J3 (Autodesk Fusion 360 design; units mm, degrees)
part number: 2026-06-01-05-43-44-829
Autodesk Fusion 360 part; units mm, degrees
sketch "Sketch1" plane through (0, 0, 0) normal (0, 0, 1) x (1, 0, 0)
  line L0 (0, 0) -> (50, 0)
  line L1 (50, 0) -> (50, 10)
  line L2 (50, 10) -> (0, 10)
  line L3 (0, 10) -> (0, 0)
  dimension "d1" = 50
  dimension "d2" = 10
  constraint horizontal L0
  constraint vertical L1
  constraint horizontal L2
  constraint vertical L3
  constraint coincident L0.start L3.end
  measures "d1" distance of L0.start L0.end
  measures "d2" distance of L0.start L2.end
extrude "Extrude1" add sketch "Sketch1" along normal blind 10
sketch "Sketch2" plane through (0, 0, 10) normal (0, 0, 1) x (-1, 0, 0)
  line L0 (0, -10) -> (0, 0)
  line L1 (0, 0) -> (-50, 0)
  line L2 (-50, 0) -> (-50, -10)
  line L3 (-50, -10) -> (0, -10)
  circle A0 centre (-5, -5) radius 4.5
  circle A1 centre (-25, -5) radius 4.5
  dimension "d5" = 9
  dimension "d6" = 9
  measures "d5" diameter of A0
  measures "d6" diameter of A1
extrude "Extrude2" cut sketch "Sketch2" against normal blind 11 contours A0 | A1
sketch "Sketch3" plane through (50, 0, 0) normal (1, 0, 0) x (0, 1, 0)
  line L0 (0, 0) -> (10, 0)
  line L1 (10, 0) -> (10, 10)
  line L2 (10, 10) -> (0, 10)
  line L3 (0, 10) -> (0, 0)
  circle A0 centre (5, 5) radius 4
  dimension "d9" = 8
  measures "d9" diameter of A0
extrude "Extrude3" cut sketch "Sketch3" against normal blind 3 contours A0
sketch "Sketch4" plane through (0, 0, 0) normal (0, -1, 0) x (1, 0, 0)
  line L0 (0, 0) -> (50, 0)
  line L1 (50, 0) -> (50, 10)
  line L2 (50, 10) -> (0, 10)
  line L3 (0, 10) -> (0, 0)
  circle A0 centre (15, 5) radius 4.5
  circle A1 centre (35, 5) radius 4.5
  dimension "d12" = 9
  dimension "d13" = 9
  measures "d12" diameter of A0
  measures "d13" diameter of A1
extrude "Extrude4" cut sketch "Sketch4" against normal blind 20 contours A0 | A1
sketch "Sketch5" plane through (0, 0, 0) normal (-1, 0, 0) x (0, -1, 0)
  line L0 (-10, 0) -> (0, 0)
  line L1 (0, 0) -> (0, 10)
  line L2 (0, 10) -> (-10, 10)
  line L3 (-10, 10) -> (-10, 0)
  circle A0 centre (-5, 5) radius 4.5
  circle A1 centre (-5, 5) radius 4
  dimension "d16" = 9
  dimension "d17" = 8
  constraint concentric A0 A1
  measures "d16" diameter of A0
  measures "d17" diameter of A1
extrude "Extrude5" add sketch "Sketch5" along normal blind 3 contours A0
